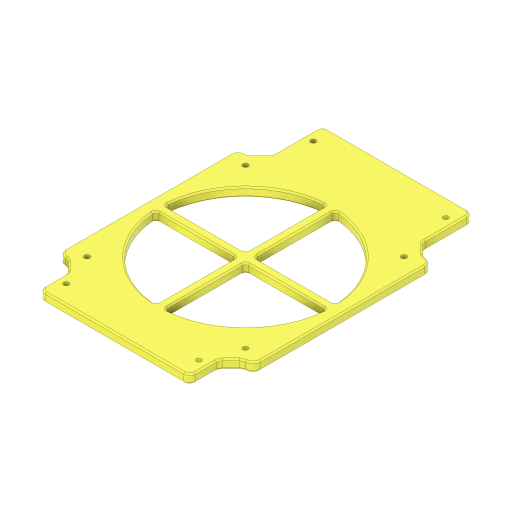
# Autodesk Inventor part: Cathode-Cover-Plate
Saved by Autodesk Inventor 2024.2 (Build 282272000, 272)
## iProperties
Created: 2023-12-01
Part Number: Cathode-Cover-Plate
Material: Generic
Document SubType Name: Modeling
Designer: kuzmin
Density: 1 g/cm^3
Appearance: Smooth - Yellow
Author: kuzmin
Autodesk Inventor part; units mm, degrees
ref_plane "YZ Plane" through (0, 0, 0) normal (1, 0, 0) x (0, 1, 0)
ref_plane "XZ Plane" through (0, 0, 0) normal (0, 1, 0) x (-1, 0, 0)
ref_plane "XY Plane" through (0, 0, 0) normal (0, 0, 1) x (1, 0, 0)
sketch "Sketch1" plane through (0, 0, 0) normal (0, 0, 1) x (1, 0, 0)
  line L0 (-94, 50) -> (94, 50)
  line L1 (94, 50) -> (94, -50)
  line L2 (94, -50) -> (-94, -50)
  line L3 (-94, -50) -> (-94, 50)
  point P0 (0, 0)
  point P1 (0, 50)
  point P2 (94, 0)
  dimension "d2" = 100
  dimension "d3" = 188
  constraints: 8 end point, 2 midpoint, 2 parallel, 1 horizontal, 1 horizontal alignment, 1 perpendicular, 1 vertical alignment
  measures "d2" distance of L0.end L1.end
  measures "d3" distance of L0.start L0.end
extrude "Extrusion1" add sketch "Sketch1" along normal blind 6
sketch "Sketch2" plane through (0, 0, 6) normal (0, 0, 1) x (1, 0, 0)
  line L0 (61.6, -59.6) -> (-47.6, -59.6) projected
  arc A0 (61.6, -59.6) -> (66.6, -54.6) centre (61.6, -54.6) ccw projected
  line L1 (-47.6, 59.6) -> (61.6, 59.6) projected
  arc A1 (-47.6, 59.6) -> (-52.6, 54.6) centre (-47.6, 54.6) ccw projected
  line L2 (66.6, 54.6) -> (66.6, -54.6) projected
  arc A2 (66.6, 54.6) -> (61.6, 59.6) centre (61.6, 54.6) ccw projected
  arc A3 (-52.6, -54.6) -> (-47.6, -59.6) centre (-47.6, -54.6) ccw projected
  line L3 (-52.6, -54.6) -> (-52.6, 54.6) projected
  circle A4 centre (7, 0) radius 56.75 projected
  circle A5 centre (59.6, 52.6) radius 1.75 projected
  circle A6 centre (59.6, -52.6) radius 1.75 projected
  circle A7 centre (-45.6, 52.6) radius 1.75 projected
  circle A8 centre (-45.6, -52.6) radius 1.75 projected
  arc A9 (66.6, 54.6) -> (61.6, 59.6) centre (61.6, 54.6) ccw projected
  line L4 (-47.6, 59.6) -> (61.6, 59.6) projected
  arc A10 (-47.6, 59.6) -> (-52.6, 54.6) centre (-47.6, 54.6) ccw projected
  line L5 (-52.6, -54.6) -> (-52.6, 54.6) projected
  arc A11 (-52.6, -54.6) -> (-47.6, -59.6) centre (-47.6, -54.6) ccw projected
  line L6 (61.6, -59.6) -> (-47.6, -59.6) projected
  arc A12 (61.6, -59.6) -> (66.6, -54.6) centre (61.6, -54.6) ccw projected
  line L7 (66.6, 54.6) -> (66.6, -54.6) projected
  point P0 (0, 0)
  point P1 (66.6, -54.6)
  point P2 (-52.6, 54.6)
extrude "Extrusion2" add sketch "Sketch2" against normal up to surface (6 mm away) contours L0 A3 L3 A1 L1 A2 L2 A0 | A4
sketch "Sketch3" plane through (0, 0, 6) normal (0, 0, 1) x (1, 0, 0)
  circle A0 centre (7, 0) radius 56.75 projected
  point P0 (0, 0)
extrude "Extrusion3" cut sketch "Sketch3" against normal through all
move faces "Move1" translate (0, -5, 0) faces at (-11.2, -59.6, 4)
move faces "Move2" translate (0, 5, 0) faces at (25.2, 59.6, 4)
sketch "Sketch7" plane through (0, 0, 6) normal (0, 0, 1) x (1, 0, 0)
  circle A0 centre (-82, -43.9615) radius 1.7
  circle A1 centre (-82, 43.9615) radius 1.7
  line L0 (-82, -43.9615) -> (-82, 43.9615) construction
  line L1 (-94, 50) -> (-94, -50) projected
  point P0 (0, 0)
  point P1 (-94, 0)
  point P2 (-82, 0)
  dimension "d32" = 87.923
  dimension "d33" = 3.4
  dimension "d34" = 12
  constraints: 2 centre point, 2 end point, 2 midpoint, 1 equal radius, 1 horizontal alignment, 1 vertical
  measures "d32" distance of L0.start L0.end
  measures "d33" diameter of A1
  measures "d34" distance between parallel lines of L1 L0
extrude "Extrusion6" cut sketch "Sketch7" against normal blind 10
chamfer "Chamfer1" distance 8.1 angle 45 4 edges at (66.6, 50, 3) (-52.6, 50, 3) (-52.6, -50, 3) (66.6, -50, 3)
fillet "Fillet1" radius 4 12 edges at (-94, 50, 3) (94, 50, 3) (94, -50, 3) (-94, -50, 3) (74.7, -50, 3) (66.6, -58.1, 3) (-52.6, -58.1, 3) (-60.7, -50, 3) (-60.7, 50, 3) (-52.6, 58.1, 3) (66.6, 58.1, 3) (74.7, 50, 3)
chamfer "Chamfer2" distance 1 angle 45 56 edges at (-56.6493, -54.0507, 6) (-52.9167, -58.1951, 6) (-51.1043, 63.1665, 6) (7, 64.6, 6) (65.1043, 63.1665, 6) (66.9167, -58.1951, 6) (70.6493, -54.0507, 6) (74.8261, -50.3045, 6) (-76.1784, -50, 6) (83.1784, -50, 6) (-92.8284, -48.8284, 6) (-94, 0, 6) (-92.8284, 48.8284, 6) (-76.1784, 50, 6) (83.1784, 50, 6) (74.8261, 50.3045, 6) (70.6493, 54.0507, 6) (66.9167, 58.1951, 6) (65.1043, -63.1665, 6) (7, -64.6, 6) (-51.1043, -63.1665, 6) (-52.9167, 58.1951, 6) (-56.6493, 54.0507, 6) (-60.8261, 50.3045, 6) (92.8284, 48.8284, 6) (94, 0, 6) (92.8284, -48.8284, 6) (-60.8261, -50.3045, 6) (7, -64.6, 0) (-51.1043, -63.1665, 0) (-52.9167, 58.1951, 0) (-56.6493, 54.0507, 0) (-60.8261, 50.3045, 0) (83.1784, 50, 0) (-76.1784, 50, 0) (92.8284, 48.8284, 0) (94, 0, 0) (92.8284, -48.8284, 0) (-76.1784, -50, 0) (83.1784, -50, 0) (-60.8261, -50.3045, 0) (-56.6493, -54.0507, 0) (-52.9167, -58.1951, 0) (-51.1043, 63.1665, 0) (7, 64.6, 0) (65.1043, 63.1665, 0) (66.9167, -58.1951, 0) (70.6493, -54.0507, 0) (74.8261, -50.3045, 0) (-92.8284, -48.8284, 0) (-94, 0, 0) (-92.8284, 48.8284, 0) (74.8261, 50.3045, 0) (70.6493, 54.0507, 0) (66.9167, 58.1951, 0) (65.1043, -63.1665, 0)
sketch "Sketch5" plane through (0, 0, 6) normal (0, 0, 1) x (1, 0, 0)
  circle A0 centre (82, -43.9615) radius 1.7
  circle A1 centre (82, 43.9615) radius 1.7
  line L0 (82, -43.9615) -> (82, 43.9615) construction
  line L1 (94, -46) -> (94, 46) projected
  point P0 (0, 0)
  point P1 (82, 0)
  point P2 (94, 0)
  dimension "d27" = 12
  dimension "d28" = 3.4
  dimension "d29" = 87.923
  constraints: 2 centre point, 2 end point, 2 midpoint, 1 equal radius, 1 horizontal alignment, 1 vertical
  measures "d27" distance between parallel lines of L1 L0
  measures "d28" diameter of A0
  measures "d29" distance of L0.start L0.end
extrude "Extrusion5" cut sketch "Sketch5" against normal through all
sketch "Sketch9" plane through (0, 0, 6) normal (0, 0, 1) x (1, 0, 0)
  circle A0 centre (7, 0) radius 56.75 projected
  line L0 (10, -56.75) -> (4, -56.75)
  line L1 (4, -56.75) -> (4, 56.75)
  line L2 (4, 56.75) -> (10, 56.75)
  line L3 (10, 56.75) -> (10, -56.75)
  line L4 (63.75, -3) -> (-49.75, -3)
  line L5 (-49.75, -3) -> (-49.75, 3)
  line L6 (-49.75, 3) -> (63.75, 3)
  line L7 (63.75, 3) -> (63.75, -3)
  point P0 (0, 0)
  point P1 (-49.75, 0)
  point P2 (7, -56.75)
  point P3 (4, -3)
  point P4 (4, -56.6706)
  point P5 (10, -56.6706)
  point P6 (10, -3)
  point P7 (63.6706, -3)
  point P8 (63.6706, 3)
  point P9 (10, 3)
  point P10 (10, 56.6706)
  point P11 (4, 56.6706)
  point P12 (4, 3)
  point P13 (-49.6706, 3)
  point P14 (-49.6706, -3)
  dimension "d37" = 6
  constraints: 16 end point, 4 parallel, 4 tangent, 3 perpendicular, 2 horizontal, 2 midpoint, 1 horizontal alignment, 1 vertical alignment
  measures "d37" distance of L0.start L0.end
extrude "Extrusion7" add sketch "Sketch9" against normal up to surface (6 mm away) contours A0 L4 L3 L6 | L3 L6 L1 A0 | L3 L4 L1 L6 | A0 L1 L4 L3 | L1 L4 A0 L6
fillet "Fillet2" radius 2 12 edges at (10, -3, 3) (4, -3, 3) (4, 3, 3) (10, 3, 3) (10, -56.6706, 3) (4, -56.6706, 3) (-49.6706, -3, 3) (-49.6706, 3, 3) (4, 56.6706, 3) (10, 56.6706, 3) (63.6706, 3, 3) (63.6706, -3, 3)
chamfer "Chamfer4" distance 1 angle 45 48 edges at (10, -29.7606, 6) (10.5858, -3.5858, 6) (36.7606, -3, 6) (62.9986, -3.6519, 6) (47.1283, -40.1283, 6) (10.6519, -55.9986, 6) (-22.7606, -3, 6) (3.4142, -3.5858, 6) (4, -29.7606, 6) (3.3481, -55.9986, 6) (-33.1283, -40.1283, 6) (-48.9986, -3.6519, 6) (-33.1283, 40.1283, 6) (3.3481, 55.9986, 6) (4, 29.7606, 6) (3.4142, 3.5858, 6) (-22.7606, 3, 6) (-48.9986, 3.6519, 6) (10.6519, 55.9986, 6) (10, 29.7606, 6) (10.5858, 3.5858, 6) (36.7606, 3, 6) (62.9986, 3.6519, 6) (47.1283, 40.1283, 6) (4, 29.7606, 0) (3.3481, 55.9986, 0) (-33.1283, 40.1283, 0) (-48.9986, 3.6519, 0) (-22.7606, 3, 0) (3.4142, 3.5858, 0) (10, 29.7606, 0) (10.5858, 3.5858, 0) (36.7606, 3, 0) (62.9986, 3.6519, 0) (47.1283, 40.1283, 0) (10.6519, 55.9986, 0) (36.7606, -3, 0) (10.5858, -3.5858, 0) (10, -29.7606, 0) (10.6519, -55.9986, 0) (47.1283, -40.1283, 0) (62.9986, -3.6519, 0) (-22.7606, -3, 0) (-48.9986, -3.6519, 0) (-33.1283, -40.1283, 0) (3.3481, -55.9986, 0) (4, -29.7606, 0) (3.4142, -3.5858, 0)
body "Solid1"
